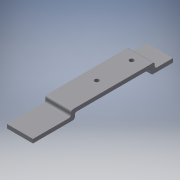
# Autodesk Inventor part: Ball screw right hand support
Saved by Autodesk Inventor 2016 (Build 200138000, 138)
## iProperties
Created: 2017-06-13
Part Number: Ball screw right hand support
Material: Generic
Document SubType Name: Modeling
Designer: m228540
Density: 1 g/cm^3
Appearance: Default
Author: m228540
Autodesk Inventor part; units mm, degrees
ref_plane "YZ Plane" through (0, 0, 0) normal (1, 0, 0) x (0, 1, 0)
ref_plane "XZ Plane" through (0, 0, 0) normal (0, 1, 0) x (-1, 0, 0)
ref_plane "XY Plane" through (0, 0, 0) normal (0, 0, 1) x (1, 0, 0)
sketch "Sketch1" plane through (0, 0, 0) normal (0, 0, 1) x (1, 0, 0)
  line L0 (-29.8485, 74.7727) -> (10.1515, 74.7727)
  line L1 (10.1515, 74.7727) -> (10.1515, -55.2273)
  line L2 (10.1515, -55.2273) -> (-29.8485, -55.2273)
  line L3 (-29.8485, -55.2273) -> (-29.8485, 74.7727)
  point P0 (0, 0)
  dimension "d0" = 40
  dimension "d1" = 130
  constraints: 8 end point, 2 parallel, 1 horizontal, 1 perpendicular
  measures "d0" distance of L1.end L2.end
  measures "d1" distance of L0.end L1.end
extrude "Extrusion1" add sketch "Sketch1" along normal blind 6
sketch "Sketch2" plane through (0, 0, 0) normal (0, 0, -1) x (-1, 0, 0)
  circle A0 centre (9.8485, 56.7727) radius 4.5 projected
  circle A1 centre (9.8485, -3.2273) radius 4.5 projected
  point P0 (0, 0)
extrude "Extrusion2" cut sketch "Sketch2" against normal through all
sketch "Sketch3" plane through (0, 0, 0) normal (0, 0, -1) x (-1, 0, 0)
  line L0 (-10.1515, 74.7727) -> (-10.1515, -55.2273) projected
  line L1 (29.8485, -55.2273) -> (29.8485, 74.7727) projected
  line L2 (-10.1515, 74.7727) -> (29.8485, 74.7727)
  line L3 (29.8485, 74.7727) -> (29.8485, 68.7727)
  line L4 (29.8485, 68.7727) -> (-10.1515, 68.7727)
  line L5 (-10.1515, 68.7727) -> (-10.1515, 74.7727)
  line L6 (-10.1515, -55.2273) -> (-10.1515, 74.7727) projected
  line L7 (29.8485, -55.2273) -> (-10.1515, -55.2273)
  line L8 (-10.1515, -55.2273) -> (-10.1515, -49.2273)
  line L9 (-10.1515, -49.2273) -> (29.8485, -49.2273)
  line L10 (29.8485, -49.2273) -> (29.8485, -55.2273)
  point P0 (0, 0)
  dimension "d6" = 6
  dimension "d7" = 6
  constraints: 16 end point, 4 parallel, 2 horizontal, 2 perpendicular, 2 point on line
  measures "d6" distance between parallel lines of L2 L4
  measures "d7" distance between parallel lines of L9 L7
extrude "Extrusion3" add sketch "Sketch3" along normal blind 3 contours L2 L1 L4 L0 | L9 L1 L7 L0
sketch "Sketch4" plane through (0, 0, -3) normal (0, 0, -1) x (-1, 0, 0)
  line L0 (-10.1515, 68.7727) -> (29.8485, 68.7727) projected
  line L1 (-10.1515, 68.7727) -> (29.8485, 68.7727)
  line L2 (29.8485, 68.7727) -> (29.8485, 102.7727)
  line L3 (29.8485, 102.7727) -> (-10.1515, 102.7727)
  line L4 (-10.1515, 102.7727) -> (-10.1515, 68.7727)
  line L5 (29.8485, -49.2273) -> (-10.1515, -49.2273) projected
  line L6 (29.8485, -49.2273) -> (-10.1515, -49.2273)
  line L7 (-10.1515, -49.2273) -> (-10.1515, -114.2273)
  line L8 (-10.1515, -114.2273) -> (29.8485, -114.2273)
  line L9 (29.8485, -114.2273) -> (29.8485, -49.2273)
  point P0 (0, 0)
  dimension "d10" = 34
  dimension "d11" = 65
  dimension "d12" = 40
  dimension "d13" = 40
  constraints: 16 end point, 4 parallel, 2 horizontal, 2 perpendicular
  measures "d10" distance of L1.end L2.end
  measures "d11" distance of L8.end L5.start
  measures "d12" distance of L7.end L8.end
  measures "d13" distance of L2.end L3.end
extrude "Extrusion4" add sketch "Sketch4" along normal blind 6
fillet "Fillet1" radius 3 8 edges at (-9.8485, 68.7727, 0) (-9.8485, 68.7727, -9) (-9.8485, 74.7727, -3) (-9.8485, 74.7727, 6) (-9.8485, -49.2273, 0) (-9.8485, -49.2273, -9) (-9.8485, -55.2273, -3) (-9.8485, -55.2273, 6)
sketch "Sketch5" plane through (0, 0, -9) normal (0, 0, -1) x (-1, 0, 0)
  circle A0 centre (11.3485, 91.2727) radius 4
  circle A1 centre (-2.6515, 91.2727) radius 4
  circle A2 centre (-2.6515, 91.2727) radius 4
  circle A3 centre (11.3485, 91.2727) radius 4
  circle A4 centre (-2.6515, 91.2727) radius 4
  circle A5 centre (11.3485, 91.2727) radius 4
  circle A6 centre (7.3485, -80.7273) radius 4
  circle A7 centre (7.3483, -96.165) radius 4
  point P0 (0, 0)
extrude "Extrusion5" cut sketch "Sketch5" against normal through all
body "Solid1"
